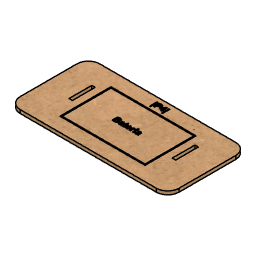
P4 (Autodesk Fusion 360 design; units mm, degrees)
Autodesk Fusion 360 part; units mm, degrees
sketch "Esboço1" plane through (0, 0, 0) normal (0, 1, 0) x (1, 0, 0)
  line L0 (-2, 0) -> (118, 0)
  line L1 (128, 10) -> (128, 60)
  line L2 (118, 70) -> (-2, 70)
  line L3 (-12, 60) -> (-12, 10)
  arc A0 (-2, 70) -> (-12, 60) centre (-2, 60) ccw
  arc A1 (128, 60) -> (118, 70) centre (118, 60) ccw
  arc A2 (-12, 10) -> (-2, 0) centre (-2, 10) ccw
  arc A3 (118, 0) -> (128, 10) centre (118, 10) ccw
  line L4 (11, 50) -> (14, 50)
  line L5 (14, 50) -> (14, 30)
  line L6 (14, 30) -> (11, 30)
  line L7 (11, 30) -> (11, 50)
  line L8 (102, 50) -> (105, 50)
  line L9 (105, 50) -> (105, 30)
  line L10 (105, 30) -> (102, 30)
  line L11 (102, 30) -> (102, 50)
  dimension "d1" = 10
  dimension "d2" = 10
  dimension "d3" = 10
  dimension "d4" = 10
  dimension "d5" = 23
  dimension "d6" = 3
  dimension "d7" = 23
  dimension "d8" = 3
  dimension "d9" = 140
  dimension "d11" = 70
  dimension "d12" = 20
  dimension "d13" = 20
  dimension "d14" = 20
  dimension "d15" = 20
  constraint horizontal L0
  constraint vertical L1
  constraint horizontal L2
  constraint vertical L3
  constraint tangent L2 A0
  constraint tangent L3 A0
  constraint tangent L1 A1
  constraint tangent L2 A1
  constraint tangent L0 A2
  constraint tangent L3 A2
  constraint tangent L0 A3
  constraint tangent L1 A3
  constraint horizontal L4
  constraint vertical L5
  constraint horizontal L6
  constraint vertical L7
  constraint horizontal L8
  constraint vertical L9
  constraint horizontal L10
  constraint vertical L11
  measures "d1" radius of A0
  measures "d2" radius of A1
  measures "d3" radius of A2
  measures "d4" radius of A3
  measures "d5" distance of L3 L7
  measures "d6" distance of L4.start L4.end
  measures "d7" distance of L1 L9
  measures "d8" distance of L8.start L8.end
  measures "d9" distance of L1 L3
  measures "d11" distance of L0 L2
  measures "d12" distance of L4.end L5.end
  measures "d13" distance of L8.end L9.end
  measures "d14" distance of L2 L4
  measures "d15" distance of L2 L8
extrude "Extrusão1" add sketch "Esboço1" along normal blind 3
sketch "Esboço2" plane through (0, 3, 0) normal (0, 1, 0) x (-1, 0, 0)
  line L0 (-14, -30) -> (-11, -30)
  line L1 (-11, -30) -> (-11, -50)
  line L2 (-11, -50) -> (-14, -50)
  line L3 (-14, -50) -> (-14, -30)
  line L4 (-105, -30) -> (-102, -30)
  line L5 (-102, -30) -> (-102, -50)
  line L6 (-102, -50) -> (-105, -50)
  line L7 (-105, -50) -> (-105, -30)
  arc A0 (-118, 0) -> (-128, -10) centre (-118, -10) ccw
  line L8 (-128, -10) -> (-128, -60)
  arc A1 (-128, -60) -> (-118, -70) centre (-118, -60) ccw
  line L9 (-118, -70) -> (2, -70)
  arc A2 (2, -70) -> (12, -60) centre (2, -60) ccw
  line L10 (12, -60) -> (12, -10)
  arc A3 (12, -10) -> (2, 0) centre (2, -10) ccw
  line L11 (2, 0) -> (-118, 0)
  line L12 (-20.5, -57.5) -> (-95.5, -57.5) construction
  line L13 (-95.5, -57.5) -> (-95.5, -69.9815) construction
  line L14 (-95.5, -69.9815) -> (-20.5, -69.9815) construction
  line L15 (-20.5, -69.9815) -> (-20.5, -57.5) construction
  line L16 (-20.5, -57.5) -> (-95.5, -57.5)
  line L17 (-95.5, -57.5) -> (-95.5, -12.5)
  line L18 (-95.5, -12.5) -> (-20.5, -12.5)
  line L19 (-20.5, -12.5) -> (-20.5, -57.5)
  line L20 (-21.5, -56.5) -> (-94.5, -56.5)
  line L21 (-94.5, -56.5) -> (-94.5, -13.5)
  line L22 (-94.5, -13.5) -> (-21.5, -13.5)
  line L23 (-21.5, -13.5) -> (-21.5, -56.5)
  line L24 (-21.5, -13.5) -> (-94.5, -13.5) construction
  line L25 (-94.5, -13.5) -> (-94.5, -56.5) construction
  line L26 (-94.5, -56.5) -> (-21.5, -56.5) construction
  line L27 (-21.5, -56.5) -> (-21.5, -13.5) construction
  dimension "d18" = 5
  dimension "d19" = 75
  dimension "d20" = 45
  dimension "d21" = 32.5
  dimension "d23" = 1
  dimension "d24" = 1
  dimension "d25" = 1
  dimension "d26" = 1
  dimension "d27" = 5
  dimension "d30" = 12.5
  text T0 "|P4|" font "Arial" height 5 bold align centre middle in box 75 x 12.4815 at (-20.5, -57.5) x (-1, 0) y (0, -1) spacing 1
  text T1 "Bateria" font "Arial" height 5 bold align centre middle in box 73 x 43 at (-21.5, -13.5) x (-1, 0) y (0, -1) spacing 1
  constraint horizontal L16
  constraint vertical L17
  constraint horizontal L18
  constraint vertical L19
  constraint coincident L12.start
  constraint horizontal L20
  constraint vertical L21
  constraint horizontal L22
  constraint vertical L23
  constraint coincident L21.end
  constraint coincident L20.start
  measures "d19" distance of L17.end L18.end
  measures "d20" distance of L12.start L18.end
  measures "d21" distance of L10 L19
  measures "d23" distance of L17 L21
  measures "d24" distance of L16 L20
  measures "d25" distance of L19 L23
  measures "d26" distance of L18 L22
  measures "d30" distance of L11 L18
extrude "Extrusão2" cut sketch "Esboço2" sketch "Esboço2" against normal blind 1 contours L16 L17 L18 L19 of sketch 2 text T1 T0
